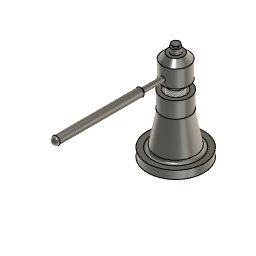
Sketch32_Final v0 (Autodesk Fusion 360 design; units mm, degrees)
Autodesk Fusion 360 part; units mm, degrees
sketch "Sketch1" plane through (0, 0, 0) normal (0, 1, 0) x (1, 0, 0)
  line L0 (49.5826, 0) -> (70, 0)
  line L1 (70, 0) -> (70, -20)
  line L2 (49.5826, 0) -> (50, 0)
  line L3 (56.5584, -20) -> (70, -20)
  line L4 (0, 0) -> (0, -3)
  line L5 (25, -145) -> (35, -145)
  line L6 (35, -145) -> (35, -105)
  line L7 (25, -145) -> (25, -105)
  line L8 (35, -105) -> (25, -105)
  line L9 (25, -105) -> (33, -105)
  line L10 (33, -105) -> (48.7138, -26.4311)
  line L11 (0, 0) -> (0, -3)
  line L12 (33, -105) -> (25, -105)
  line L13 (50, 0) -> (49.5826, 0)
  line L14 (25, -105) -> (41.5143, -3)
  line L15 (41.5143, -3) -> (45, -3)
  arc A0 (45, -3) -> (49.5826, 0) centre (45, 2) ccw
  arc A1 (56.5584, -20) -> (48.7138, -26.4311) centre (56.5584, -28) ccw
  dimension "d1" = 70
  dimension "d2" = 20
  dimension "d3" = 50
  dimension "d10" = 40
  dimension "d12" = 3
  dimension "d14" = 5
  dimension "d15" = 8
  constraint horizontal L0
  constraint perpendicular L0 L1
  constraint coincident L4.start L11.start
  constraint perpendicular L1 L2
  constraint perpendicular L1 L3
  constraint perpendicular L0 L4
  constraint perpendicular L4 L5
  constraint perpendicular L5 L6
  constraint perpendicular L7 L8
  constraint perpendicular L7 L9
  constraint perpendicular L2 L11
  constraint perpendicular L7 L12
  constraint tangent L15 A0
  constraint tangent L10 A1
  constraint tangent L3 A1
  measures "d1" distance of L4.start L0.end
  measures "d2" distance of L0.end L1.end
  measures "d3" distance of L4.start L2.end
  measures "d10" distance of L5.end L6.end
  measures "d12" distance of L4.start L4.end
  measures "d14" radius of A0
  measures "d15" radius of A1
revolve "Revolve1" add sketch "Sketch1" angle 360 about axis through (0, 0, 1.75) along (0, 0, 1) makes body 1
copy_body "Body->Comp1" bodies 1 removing the originals makes body 2 in component "GaugeBody"
sketch "Sketch2" plane through (0, 0, 0) normal (0, 1, 0) x (1, 0, 0)
  line L0 (0, 0) -> (25, 0)
  line L1 (25, 0) -> (25, -20)
  line L2 (25, -45) -> (25, -40)
  line L3 (30, -35) -> (40, -35)
  line L4 (45, -30) -> (45, -30)
  line L5 (40, -25) -> (30, -25)
  arc A0 (30, -35) -> (25, -40) centre (30, -40) ccw
  arc A1 (40, -35) -> (45, -30) centre (40, -30) ccw
  arc A2 (45, -30) -> (40, -25) centre (40, -30) ccw
  line L6 (0, 0) -> (19, 0)
  line L7 (19, 0) -> (19, -45)
  line L8 (19, -45) -> (25, -45)
  arc A3 (25, -20) -> (30, -25) centre (30, -20) ccw
  point P0 (25, -35)
  point P1 (0, -35)
  point P2 (45, -35)
  point P3 (45, -25)
  dimension "d17" = 25
  dimension "d18" = 45
  dimension "d19" = 10
  dimension "d20" = 45
  dimension "d21" = 10
  dimension "d22" = 5
  dimension "d23" = 5
  dimension "d24" = 5
  dimension "d25" = 19
  dimension "d26" = 5
  constraint coincident L0.start L6.start
  constraint horizontal L0
  constraint perpendicular L0 L1
  constraint parallel L1 L2
  constraint perpendicular L1 L3
  constraint perpendicular L1 L5
  constraint coincident P0 L2
  constraint coincident P1 L3
  constraint tangent L2 A0
  constraint tangent L3 A0
  constraint coincident P2 L3
  constraint tangent L3 A1
  constraint coincident P3 L4
  constraint coincident P3 L5
  constraint tangent L5 A2
  constraint parallel L0 L6
  constraint perpendicular L6 L7
  constraint coincident L2.start L1
  constraint tangent L1 A3
  constraint tangent L5 A3
  measures "d17" distance of L0.start L0.end
  measures "d18" distance of L0.end L2.start
  measures "d19" distance of L2.start P0
  measures "d20" distance of P1 P2
  measures "d21" distance of P2 P3
  measures "d22" radius of A0
  measures "d23" radius of A1
  measures "d24" radius of A2
  measures "d25" distance of L0.start L6.end
  measures "d26" radius of A3
revolve "Revolve2" add sketch "Sketch2" angle 360 about axis through (0, 0, 1.75) along (0, 0, 1) separate body makes body 3
copy_body "Body->Comp2" bodies 3 removing the originals makes body 4 in component "Nut"
sketch "Sketch3" plane through (0, 0, 0) normal (0, 1, 0) x (1, 0, 0)
  line L0 (0, 0) -> (19, 0)
  line L1 (19, 0) -> (19, -227)
  line L2 (0, -227) -> (0, -157)
  line L3 (0, -157) -> (19, -157)
  line L4 (32.5, -213.5) -> (32.5, -170.5)
  line L5 (0, -157) -> (0, -192)
  line L6 (0, -227) -> (19, -227)
  line L7 (19, -227) -> (32.5, -213.5)
  line L8 (19, -227) -> (39.0391, -227) construction
  line L9 (32.5, -170.5) -> (19, -157)
  line L10 (0, 0) -> (0, -157)
  line L11 (0, -227) -> (11, -227)
  line L12 (11, -227) -> (11, -240)
  line L13 (11, -240) -> (0, -240)
  line L14 (0, -240) -> (0, -227)
  dimension "d28" = 19
  dimension "d33" = 35
  dimension "d35" = 45
  dimension "d37" = 11
  constraint coincident L0.start L10.start
  constraint horizontal L0
  constraint perpendicular L0 L1
  constraint perpendicular L1 L3
  constraint perpendicular L3 L5
  constraint perpendicular L4 L6
  constraint horizontal L8
  constraint coincident L1 L3.end
  constraint perpendicular L3 L10
  constraint perpendicular L2 L11
  constraint perpendicular L11 L12
  constraint perpendicular L12 L13
  constraint perpendicular L11 L14
  measures "d28" distance of L0.start L0.end
  measures "d33" distance of L2.end L5.end
  measures "d35" angle of L7 L8
  measures "d37" distance of L2.start L11.end
revolve "Revolve3" add sketch "Sketch3" angle 360 about axis through (0, 0, 0) along (0, 0, 1) separate body makes body 5
thread "Thread1" "ISO Metric profile 38.0 M38x1.5 6g" major diameter 37.85 minor diameter 36.1319 pitch 1.5 angle 60 resizes the face on face at (18.9764, -0.9471, 52.3333) on bodies 5
hole "Hole1" at (0, -32.5, 185.5777) direction (0, 1, 0) diameter 12 depth 10 tip angle 180 bodies 5
sketch "Sketch5" plane through (0, 0, 240) normal (0, 0, 1) x (-1, 0, 0)
  circle A0 centre (0, 0) radius 11
  circle A1 centre (0, 0) radius 6
  dimension "d47" = 12
  constraint concentric A0 A1
  measures "d47" diameter of A1
extrude "Extrude1" cut sketch "Sketch5" against normal blind 30 contours A1 bodies 5
copy_body "Body->Comp3" bodies 5 removing the originals makes body 6 in component "Screw"
thread "Thread1'" "ISO Metric profile 38.0 M38x1.5 6H" major diameter 38.2083 minor diameter 36.5262 pitch 1.5 angle 60 resizes the face on face at (18.9764, -0.9471, 15) on bodies 4 in component "Nut"
sketch "Sketch6" plane through (0, 0, 0) normal (0, 1, 0) x (1, 0, 0)
  line L0 (0, 0) -> (6, 0)
  line L1 (6, 0) -> (6, -30)
  line L2 (6, -30) -> (9.4641, -36)
  line L3 (6, -30) -> (29.2412, -30) construction
  line L4 (0, -30) -> (0, -36)
  line L5 (0, -36) -> (9.4641, -36)
  line L6 (0, -30) -> (0, 0)
  dimension "d50" = 6
  dimension "d51" = 30
  dimension "d52" = 60
  dimension "d53" = 6
  constraint coincident L0.start L6.end
  constraint horizontal L0
  constraint perpendicular L0 L1
  constraint horizontal L3
  constraint vertical L4
  constraint perpendicular L4 L5
  constraint perpendicular L0 L6
  measures "d50" distance of L0.start L0.end
  measures "d51" distance of L0.end L1.end
  measures "d52" angle of L2 L3
  measures "d53" distance of L4.start L4.end
revolve "Revolve4" add sketch "Sketch6" angle 360 about axis through (0, 0, 30) along (0, 0, -1) separate body makes body 7
sketch "Sketch7" plane through (0, 0, 0) normal (0, 1, 0) x (1, 0, 0)
  line L0 (0, 0) -> (0, -6)
  line L1 (0, -6) -> (62, -6)
  line L2 (0, 0) -> (275, 0)
  line L3 (275, 0) -> (275, -10)
  line L4 (62, -6) -> (66, -10)
  line L5 (62, -6) -> (93.901, -6) construction
  line L6 (275, -10) -> (66, -10)
  line L7 (275, 0) -> (285, 0)
  arc A0 (275, -10) -> (285, 0) centre (275, 0) ccw
  dimension "d55" = 6
  dimension "d56" = 62
  dimension "d57" = 275
  dimension "d58" = 10
  dimension "d59" = 45
  constraint coincident L0.start L2.start
  constraint vertical L0
  constraint perpendicular L0 L1
  constraint perpendicular L0 L2
  constraint perpendicular L2 L3
  constraint horizontal L5
  constraint perpendicular L3 L6
  constraint perpendicular L3 L7
  constraint tangent L6 A0
  measures "d55" distance of L0.start L0.end
  measures "d56" distance of L0.end L1.end
  measures "d57" distance of L0.start L2.end
  measures "d58" distance of L2.end L3.end
  measures "d59" angle of L4 L5
revolve "Revolve5" add sketch "Sketch7" angle 360 about axis through (0, 0, 0) along (1, 0, 0) separate body contours L0 L1 L2 L3 L4 L6 makes body 8
revolve "Revolve6" add sketch "Sketch7" angle 360 about axis through (275, 0, 0) along (1, 0, 0) contours L3 L7 A0 bodies 8
copy_body "Body->Comp4" bodies 7 removing the originals makes body 9 in component "screws"
copy_body "Body->Comp5" bodies 8 removing the originals makes body 10 in component "TommyBar"
component "GaugeBody" placed x (1, 0, 0) y (0, 1, 0) z (0, 0, 1) at (120.7055, 147.9644, 27.259)
component "Nut" placed x (1, 0, 0) y (0, 1, 0) z (0, 0, 1) at (120.7055, 147.9644, 33.6901)
component "Screw" placed x (1, 0, 0) y (0, 1, 0) z (0, 0, 1) at (120.7055, 147.9644, 25.2276)
component "screws" placed x (1, 0, 0) y (0, 1, 0) z (0, 0, 1) at (120.7055, 147.9644, 235.2276)
component "TommyBar" placed x (0, -1, 0) y (0, 0, -1) z (1, 0, 0) at (120.7055, 125.4644, 210.8053)
named bodies: "Nut", "Screw", "screws", "TommyBar"
